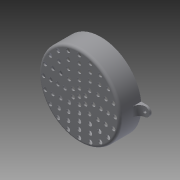
# Autodesk Inventor part: raspi-holder-top-speaker
Saved by Autodesk Inventor 2014 (Build 180170000, 170)
## iProperties
Created: 2017-08-16
Part Number: raspi-holder-top-speaker
Material: 一般
Document SubType Name: Modeling
Designer: hide
Density: 1 g/cm^3
Appearance: 既定
Author: hide
Autodesk Inventor part; units mm, degrees
note: some values were not read from the file. Chosen so that the rebuilt part matches the saved one: sketch regions of "押し出し4"; arc direction of "押し出し4".
ref_plane "YZ Plane" through (0, 0, 0) normal (1, 0, 0) x (0, 1, 0)
ref_plane "XZ Plane" through (0, 0, 0) normal (0, 1, 0) x (-1, 0, 0)
ref_plane "XY Plane" through (0, 0, 0) normal (0, 0, 1) x (1, 0, 0)
sketch "スケッチ1" plane through (0, 0, 0) normal (0, 1, 0) x (-1, 0, 0)
  circle A0 centre (0, 0) radius 30
  dimension "d0" = 60
  constraints: 1 centre point, 1 coincident
  measures "d0" diameter of A0
extrude "押し出し1" add sketch "スケッチ1" along normal blind 16
sketch "スケッチ2" plane through (0, 16, 0) normal (0, 1, 0) x (1, 0, 0)
  circle A0 centre (0, 0) radius 30 projected
  circle A1 centre (0, 0) radius 29
  dimension "d3" = 58
  constraints: 1 centre point, 1 coincident
  measures "d3" diameter of A1
extrude "押し出し2" cut sketch "スケッチ2" against normal blind 15 contours A1
sketch "スケッチ3" plane through (0, 0, 0) normal (0, -1, 0) x (1, 0, 0)
  circle A0 centre (0, 0) radius 30 projected
  circle A1 centre (0, 26.5) radius 1.5
  circle A2 centre (0, 21.2) radius 1.5
  circle A3 centre (0, 15.9) radius 1.5
  circle A4 centre (0, 10.6) radius 1.5
  circle A5 centre (0, 0) radius 1.5
  circle A6 centre (0, 5.3) radius 1.5
  circle A7 centre (-8.189, 25.203) radius 1.5
  circle A8 centre (-15.5763, 21.439) radius 1.5
  circle A9 centre (-21.439, 15.5763) radius 1.5
  circle A10 centre (-25.203, 8.189) radius 1.5
  circle A11 centre (-26.5, 0) radius 1.5
  circle A12 centre (-25.203, -8.189) radius 1.5
  circle A13 centre (-21.439, -15.5763) radius 1.5
  circle A14 centre (-15.5763, -21.439) radius 1.5
  circle A15 centre (-8.189, -25.203) radius 1.5
  circle A16 centre (0, -26.5) radius 1.5
  circle A17 centre (8.189, -25.203) radius 1.5
  circle A18 centre (15.5763, -21.439) radius 1.5
  circle A19 centre (21.439, -15.5763) radius 1.5
  circle A20 centre (25.203, -8.189) radius 1.5
  circle A21 centre (26.5, 0) radius 1.5
  circle A22 centre (25.203, 8.189) radius 1.5
  circle A23 centre (21.439, 15.5763) radius 1.5
  circle A24 centre (15.5763, 21.439) radius 1.5
  circle A25 centre (8.189, 25.203) radius 1.5
  circle A26 centre (-8.1129, 19.5862) radius 1.5
  circle A27 centre (-14.9907, 14.9907) radius 1.5
  circle A28 centre (-19.5862, 8.1129) radius 1.5
  circle A29 centre (-21.2, 0) radius 1.5
  circle A30 centre (-19.5862, -8.1129) radius 1.5
  circle A31 centre (-14.9907, -14.9907) radius 1.5
  circle A32 centre (-8.1129, -19.5862) radius 1.5
  circle A33 centre (0, -21.2) radius 1.5
  circle A34 centre (8.1129, -19.5862) radius 1.5
  circle A35 centre (14.9907, -14.9907) radius 1.5
  circle A36 centre (19.5862, -8.1129) radius 1.5
  circle A37 centre (21.2, 0) radius 1.5
  circle A38 centre (19.5862, 8.1129) radius 1.5
  circle A39 centre (14.9907, 14.9907) radius 1.5
  circle A40 centre (8.1129, 19.5862) radius 1.5
  circle A41 centre (-7.95, 13.7698) radius 1.5
  circle A42 centre (-13.7698, 7.95) radius 1.5
  circle A43 centre (-15.9, 0) radius 1.5
  circle A44 centre (-13.7698, -7.95) radius 1.5
  circle A45 centre (-7.95, -13.7698) radius 1.5
  circle A46 centre (0, -15.9) radius 1.5
  circle A47 centre (7.95, -13.7698) radius 1.5
  circle A48 centre (13.7698, -7.95) radius 1.5
  circle A49 centre (15.9, 0) radius 1.5
  circle A50 centre (13.7698, 7.95) radius 1.5
  circle A51 centre (7.95, 13.7698) radius 1.5
  circle A52 centre (-7.4953, 7.4953) radius 1.5
  circle A53 centre (-10.6, 0) radius 1.5
  circle A54 centre (-7.4953, -7.4953) radius 1.5
  circle A55 centre (0, -10.6) radius 1.5
  circle A56 centre (7.4953, -7.4953) radius 1.5
  circle A57 centre (10.6, 0) radius 1.5
  circle A58 centre (7.4953, 7.4953) radius 1.5
  circle A59 centre (-4.5899, 2.65) radius 1.5
  circle A60 centre (-4.5899, -2.65) radius 1.5
  circle A61 centre (0, -5.3) radius 1.5
  circle A62 centre (4.5899, -2.65) radius 1.5
  circle A63 centre (4.5899, 2.65) radius 1.5
  dimension "d6" = 3
  dimension "d7" = 3
  dimension "d8" = 3
  dimension "d9" = 3
  dimension "d10" = 3
  dimension "d11" = 3
  dimension "d12" = 0
  dimension "d13" = 0
  dimension "d14" = 0
  dimension "d15" = 0
  dimension "d16" = 0
  dimension "d17" = 5.3
  dimension "d18" = 5.3
  dimension "d19" = 5.3
  dimension "d20" = 5.3
  dimension "d21" = 5.3
  dimension "d24" = 360
  dimension "d28" = 360
  dimension "d32" = 360
  dimension "d36" = 360
  dimension "d40" = 360
  constraints: 63 centre point, 1 coincident, 129 other
  measures "d6" diameter of A5
  measures "d7" diameter of A6
  measures "d8" diameter of A4
  measures "d9" diameter of A3
  measures "d10" diameter of A2
  measures "d11" diameter of A1
  measures "d12" horizontal distance of A6.centre A0.centre
  measures "d13" horizontal distance of A0.centre A4.centre
  measures "d14" horizontal distance of A0.centre A3.centre
  measures "d15" horizontal distance of A0.centre A2.centre
  measures "d16" horizontal distance of A0.centre A1.centre
  measures "d17" distance of A0.centre A6.centre
  measures "d18" distance of A6.centre A4.centre
  measures "d19" distance of A4.centre A3.centre
  measures "d20" distance of A3.centre A2.centre
  measures "d21" distance of A2.centre A1.centre
extrude "押し出し3" cut sketch "スケッチ3" against normal blind 15 contours A1 | A2 | A3 | A4 | A5 | A6 | A7 | A8 | A9 | A10 | A11 | A12 | A13 | A14 | A15 | A16 | A17 | A18 | A19 | A20 | A21 | A22 | A23 | A24 | A25 | A26 | A27 | A28 | A29 | A30 | A31 | A32 | A33 | A34 | A35 | A36 | A37 | A38 | A39 | A40 | A41 | A42 | A43 | A44 | A45 | A46 | A47 | A48 | A49 | A50 | A51 | A52 | A53 | A54 | A55 | A56 | A57 | A58 | A59 | A60 | A61 | A62 | A63
sketch "スケッチ4" plane through (0, 16, 0) normal (0, 1, 0) x (1, 0, 0)
  circle A0 centre (0, 0) radius 29 projected
  circle A1 centre (-34, 0) radius 3.5
  circle A2 centre (34, 0) radius 3.5
  line L0 (-34, 3.5) -> (-29.1988, 3.5)
  line L1 (-29.1988, 3.5) -> (-29.1988, -3.5)
  line L2 (-29.1988, -3.5) -> (-34, -3.5)
  line L3 (34, 3.5) -> (29.542, 3.5)
  line L4 (29.542, 3.5) -> (29.542, -3.5)
  line L5 (29.542, -3.5) -> (34, -3.5)
  circle A3 centre (-34, 0) radius 1.1
  circle A4 centre (34, 0) radius 1.1
  line L6 (-34, -3.5) -> (-34, -1.1)
  line L7 (-34, 1.1) -> (-34, 3.5)
  line L8 (34, -3.5) -> (34, -1.1)
  line L9 (34, 1.1) -> (34, 3.5)
  dimension "d47" = 7
  dimension "d49" = 7
  dimension "d44" = 34
  dimension "d45" = 34
  dimension "d46" = 7
  dimension "d48" = 0
  dimension "d50" = 7
  dimension "d52" = 2.2
  dimension "d53" = 2.2
  constraints: 20 end point, 6 parallel, 4 point on circle, 2 centre point, 2 coincident, 2 horizontal, 2 perpendicular, 2 vertical alignment, 4 other
  measures "d44" distance of A0.centre A3.centre
  measures "d45" distance of A0.centre point (34, 0)
  measures "d46" distance of L2.end L0.start
  measures "d48" vertical extent of L2
  measures "d50" distance of L5.end L3.start
  measures "d52" diameter of A4
  measures "d53" diameter of A3
extrude "押し出し4" add sketch "スケッチ4" against normal blind 1.5 contours A1 L6 A3 L7 | A1 L0 L1 L2 | L7 A3 L6 A1 | A2 L8 A4 L9 | L9 A4 L8 A2 | A2 L5 L4 L3
fillet "フィレット1" radius 5 3 edges at (30, 14.5, 0) (-29.9487, 14.5, -1.753) (-29.9487, 14.5, 1.753)
fillet "フィレット2" radius 1 1 edges at (-29, 1, 0)
fillet "フィレット3" radius 2 1 edges at (30, 0, 0)
equation "\"d7\" = d6"
equation "\"d8\" = d7"
equation "\"d9\" = d7"
equation "\"d10\" = d7"
equation "\"d11\" = d7"
equation "\"d18\" = d17"
equation "\"d19\" = d18"
equation "\"d20\" = d19"
equation "\"d21\" = d20"
equation "\"d47\" = d46"
equation "\"d49\" = d47"
equation "\"d45\" = d44"
equation "\"d50\" = d49"
equation "\"d53\" = d52"
